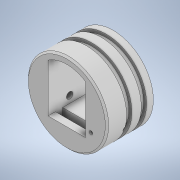
# Autodesk Inventor part: LEDSlideHolder
Saved by Autodesk Inventor 2020 (Build 240168000, 168)
## iProperties
Created: 2019-09-15
Part Number: LEDSlideHolder
Material: Generic
Document SubType Name: Modeling
Designer: strom
Density: 1 g/cm^3
Appearance: Default
Mass: 103.102 g
Surface Area: 216.515 cm^2
Volume: 103.102 cm^3
Author: strom
Autodesk Inventor part; units mm, degrees
ref_plane "YZ Plane" through (0, 0, 0) normal (1, 0, 0) x (0, 1, 0)
sketch "Sketch1" plane through (0, 0, 0) normal (0, 0, 1) x (1, 0, 0)
  circle A0 centre (0, 0) radius 37.7444
  dimension "d0" = 75.4888
  constraints: 1 centre point, 1 coincident
  measures "d0" diameter of A0
extrude "Extrusion1" add sketch "Sketch1" along normal blind 38.1
sketch "Sketch2" plane through (0, 0, 0) normal (0, 0, -1) x (-1, 0, 0)
  circle A0 centre (0, 0) radius 31.7754
  line L0 (-17.653, 26.4206) -> (-17.653, -26.4206)
  line L1 (17.653, 26.4206) -> (17.653, -26.4206)
  line L2 (-96.4115, 0) -> (174.9509, 0)
  line L3 (0, -219.9579) -> (0, 88.8884)
  line L4 (-17.653, -19.05) -> (17.653, -19.05)
  dimension "d3" = 63.5508
  dimension "d4" = 35.306
  dimension "d5" = 19.05
  constraints: 10 end point, 4 point on circle, 2 point on line, 2 vertical, 1 centre point, 1 coincident, 1 horizontal, 1 parallel, 1 perpendicular, 5 other
  measures "d3" diameter of A0
  measures "d4" distance between parallel lines of L1 L0
  measures "d5" distance between parallel lines of L4 L2
extrude "Extrusion2" cut sketch "Sketch2" against normal through all contours L1 L2 L3 A0 | L1 L4 L3 L2 | L3 L2 L0 A0 | L3 L4 L0 L2
ref_plane "Work Plane1" through (0, 0, 0) normal (-1, 0, 0) x (0, 0, 1)
sketch "Sketch3" plane through (0, 0, 0) normal (-1, 0, 0) x (0, 0, 1)
  circle A0 centre (17.78, -12.446) radius 3.048
  line L0 (38.1, 26.4206) -> (38.1, -19.05) projected
  line L1 (0, 26.4206) -> (38.1, 26.4206) projected
  line L2 (0, -19.05) -> (0, 26.4206) projected
  line L3 (0, -19.05) -> (38.1, -19.05) projected
  circle A1 centre (27.94, -12.446) radius 3.048
  point P0 (0, 0)
  dimension "d8" = 6.096
  dimension "d10" = 6.096
  dimension "d11" = 10.16
  dimension "d12" = 10.16
  dimension "d13" = 6.604
  constraints: 2 centre point, 1 horizontal alignment
  measures "d8" diameter of A0
  measures "d10" diameter of A1
  measures "d11" distance of A1.centre A0.centre
  measures "d12" distance from line of L0 A1.centre
  measures "d13" distance from line of A0.centre L3
extrude "Extrusion3" cut sketch "Sketch3" against normal through all both and the other way through all contours A0
sketch "Sketch4" plane through (0, 0, 0) normal (0, 0, -1) x (-1, 0, 0)
  line L0 (-17.653, -9.398) -> (-36.5557, -9.398) projected
  line L1 (-17.653, -15.494) -> (-34.4177, -15.494) projected
  line L2 (36.5557, -9.398) -> (17.653, -9.398) projected
  line L3 (34.4177, -15.494) -> (17.653, -15.494) projected
  line L4 (-17.653, -19.05) -> (-17.653, 26.4206) projected
  line L5 (17.653, -19.05) -> (-17.653, -19.05) projected
  line L6 (17.653, 26.4206) -> (17.653, -19.05) projected
  arc A0 (17.653, 26.4206) -> (-17.653, 26.4206) centre (0, 0) ccw projected
  circle A1 centre (-22.733, -12.446) radius 1.651
  dimension "d17" = 3.048
  dimension "d18" = 3.302
  dimension "d19" = 5.08
  constraints: 1 centre point
  measures "d17" distance from line of L0 A1.centre
  measures "d18" diameter of A1
  measures "d19" distance from line of A1.centre L4
extrude "Extrusion4" cut sketch "Sketch4" against normal through all contours A1
sketch "Sketch6" plane through (0, 0, 0) normal (0, 1, 0) x (-1, 0, 0)
  line L0 (-17.653, 20.828) -> (-35.6334, 20.828) projected
  line L1 (-17.653, 14.732) -> (-35.6334, 14.732) projected
  line L2 (35.6334, 20.828) -> (17.653, 20.828) projected
  line L3 (35.6334, 14.732) -> (17.653, 14.732) projected
  line L4 (-17.653, 38.1) -> (17.653, 38.1) projected
  line L5 (-17.653, 0) -> (-17.653, 38.1) projected
  line L6 (17.653, 0) -> (-17.653, 0) projected
  line L7 (17.653, 0) -> (17.653, 38.1) projected
  line L8 (-17.653, 0) -> (-17.653, 38.1) projected
  line L9 (17.653, 0) -> (17.653, 38.1) projected
  line L10 (-17.653, 24.384) -> (17.653, 24.384)
  line L11 (17.653, 24.384) -> (17.653, 31.242)
  line L12 (17.653, 31.242) -> (-17.653, 31.242)
  line L13 (-17.653, 31.242) -> (-17.653, 24.384)
  point P0 (0, 0)
  dimension "d23" = 6.858
  dimension "d24" = 3.556
  constraints: 8 end point, 2 parallel, 2 point on line, 1 horizontal, 1 perpendicular
  measures "d23" distance of L11.end L10.end
  measures "d24" distance between parallel lines of L10 L2
extrude "Extrusion5" cut sketch "Sketch6" against normal through all contours L12 L7 L10 L5
ref_plane "Work Plane2" through (0, 0, 14.732) normal (0, 0, -1) x (-1, 0, 0)
sketch "Sketch7" plane through (0, 0, 14.732) normal (0, 0, -1) x (-1, 0, 0)
  circle A0 centre (0, 0) radius 34.9504
  circle A1 centre (0, 0) radius 37.7444 projected
  dimension "d30" = 2.794
  constraints: 1 centre point, 1 coincident
  measures "d30" radial gap between concentric circles of A1 A0
extrude "Extrusion6" cut sketch "Sketch7" against normal blind 4.953
ref_plane "Work Plane3" through (0, 0, 5.842) normal (0, 0, -1) x (-1, 0, 0)
sketch "Sketch8" plane through (0, 0, 5.842) normal (0, 0, -1) x (-1, 0, 0)
  circle A0 centre (0, 0) radius 37.7444
  arc A1 (36.3772, -10.0667) -> (-36.3772, -10.0667) centre (0, 0) ccw projected
  circle A2 centre (0, 0) radius 34.9504
  dimension "d33" = 2.794
  constraints: 2 centre point, 2 coincident, 2 concentric
  measures "d33" radial gap between concentric circles of A2 A0
extrude "Extrusion7" cut sketch "Sketch8" along normal blind 4.953
move faces "Move1" translate (0, 0, -5.461) faces at (-24.0347, 5.2565, 0)
chamfer "Chamfer1" distance 1.5875 angle 45 1 edges at (-37.7444, 0, 38.1)
body "Solid1"
